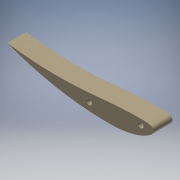
# Autodesk Inventor part: uretan_ms
Saved by Autodesk Inventor 2018 (Build 220112000, 112)
## iProperties
Created: 2018-04-20
Part Number: uretan_ms
Material: ポリエチレン、高密度
Document SubType Name: Modeling
Designer: ku_sk
Density: 0.952 g/cm^3
Appearance: ベージュ
Author: ku_sk
Autodesk Inventor part; units mm, degrees
ref_plane "YZ Plane" through (0, 0, 0) normal (1, 0, 0) x (0, 1, 0)
ref_plane "XZ Plane" through (0, 0, 0) normal (0, 1, 0) x (-1, 0, 0)
ref_plane "XY Plane" through (0, 0, 0) normal (0, 0, 1) x (1, 0, 0)
sketch "スケッチ1" plane through (0, 0, 0) normal (0, 1, 0) x (-1, 0, 0)
  arc A0 (99.4141, -32.927) -> (304.2493, 7.0592) centre (88.5018, 567.6156) ccw projected
  arc A1 (73.8469, -32.6347) -> (99.4141, -32.927) centre (91.566, 398.982) ccw projected
  arc A2 (27.3573, -24.3709) -> (73.8469, -32.6347) centre (81.048, 142.776) ccw projected
  arc A3 (0.844, -11.3484) -> (27.3573, -24.3709) centre (58.458, 72.45) ccw projected
  arc A4 (-6.1834, -4.5246) -> (0.844, -11.3484) centre (17.4, 12.732) ccw projected
  arc A5 (-1.3535, 7.5415) -> (-6.1834, -4.5246) centre (0, 0) ccw projected
  arc A6 (18.2937, 9.3227) -> (-1.3535, 7.5415) centre (18.66, -103.968) ccw projected
  arc A7 (85.069, 6.346) -> (18.2937, 9.3227) centre (20.556, -690.396) ccw projected
  arc A8 (85.069, 6.346) -> (126.1777, 2.6065) centre (1264.674, 12746.1) ccw projected
  arc A9 (126.1777, 2.6065) -> (203.1141, -0.6229) centre (198.864, 816.2039) ccw projected
  arc A10 (203.1141, -0.6229) -> (304.2493, 7.0592) centre (199.374, 718.188) ccw projected
  circle A11 centre (20, -2.2582) radius 6 projected
  circle A12 centre (130, -14.678) radius 6 projected
extrude "押し出し2" add sketch "スケッチ1" along normal mid plane 40.2
